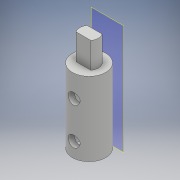
# Autodesk Inventor part: Ośka
Saved by Autodesk Inventor 2017 (Build 210142000, 142)
## iProperties
Created: 2018-08-19
Part Number: Ośka
Material: Ogólny
Document SubType Name: Modeling
Designer: Wojciech
Density: 1 g/cm^3
Appearance: Domyślna
Author: Wojciech
Autodesk Inventor part; units mm, degrees
ref_plane "YZ Plane" through (0, 0, 0) normal (1, 0, 0) x (0, 1, 0)
ref_plane "XY Plane" through (0, 0, 0) normal (0, 0, 1) x (1, 0, 0)
sketch "Szkic1" plane through (0, 0, 0) normal (0, 0, 1) x (1, 0, 0)
  circle A0 centre (0, 0) radius 4.5
  dimension "d0" = 9
  constraints: 1 centre point, 1 coincident
  measures "d0" diameter of A0
extrude "Wyciągnięcie proste1" add sketch "Szkic1" along normal blind 20
sketch "Szkic2" plane through (0, 0, 0) normal (0, 0, -1) x (-1, 0, 0)
  circle A0 centre (0, 0) radius 3
  dimension "d3" = 6
  constraints: 1 centre point, 1 coincident
  measures "d3" diameter of A0
extrude "Wyciągnięcie proste2" cut sketch "Szkic2" against normal blind 17
sketch "Szkic3" plane through (0, 0, 20) normal (0, 0, 1) x (1, 0, 0)
  circle A0 centre (0, 0) radius 2.5
  line L0 (-2, 1.5) -> (2, 1.5)
  line L1 (-2, -1.5) -> (2, -1.5)
  dimension "d6" = 5
  dimension "d7" = 1.5
  dimension "d8" = 1.5
  constraints: 4 end point, 4 point on circle, 2 horizontal, 1 centre point, 1 coincident
  measures "d6" diameter of A0
  measures "d7" distance from line of L0 point (0, 0)
  measures "d8" distance from line of L1 point (0, 0)
extrude "Wyciągnięcie proste3" add sketch "Szkic3" along normal blind 7 contours A0 L1 L0
ref_plane "Płaszczyzna konstrukcyjna1" through (0, 5, 0) normal (0, 1, 0) x (-1, 0, 0)
sketch "Szkic6" plane through (0, 5, 0) normal (0, 1, 0) x (-1, 0, 0)
  line L0 (-2, 20) -> (-2, 27) projected
  point P0 (0, 0)
  point P1 (-0.2386, 3.9929)
  point P2 (-0.2386, 13.9929)
  dimension "d12" = 10
  dimension "d13" = 4
  dimension "d14" = 1.7614
  dimension "d15" = 1.7614
  measures "d12" distance of point (-0.239, 13.993) point (-0.239, 3.993)
  measures "d13" distance of point (0, 0) point (-0.239, 3.993)
  measures "d14" distance from line of L0 point (-0.239, 3.993)
  measures "d15" distance from line of L0 point (-0.239, 13.993)
hole "Otwór1" at (0.2386, 5, 3.9929) at (0.2386, 5, 13.9929) direction (0, -1, 0) diameter 3 end through all
